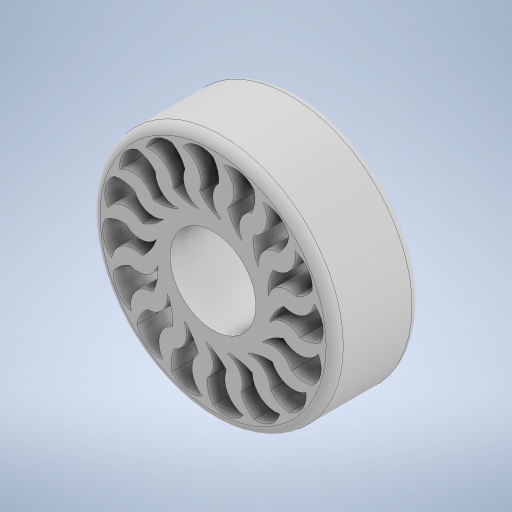
# Autodesk Inventor part: Idea1
Saved by Autodesk Inventor 2024.2 (Build 282272000, 272)
## iProperties
Created: 2025-06-20
Part Number: Idea1
Material: Generic
Document SubType Name: Modeling
Designer: Admin
Density: 1 g/cm^3
Appearance: Default
Author: Admin
Autodesk Inventor part; units mm, degrees
ref_plane "YZ Plane" through (0, 0, 0) normal (1, 0, 0) x (0, 1, 0)
ref_plane "XZ Plane" through (0, 0, 0) normal (0, 1, 0) x (-1, 0, 0)
ref_plane "XY Plane" through (0, 0, 0) normal (0, 0, 1) x (1, 0, 0)
sketch "Sketch1" plane through (0, 0, 0) normal (0, 0, 1) x (1, 0, 0)
  circle A0 centre (0, 0) radius 15
  circle A1 centre (0, 0) radius 42.5
  line L0 (2.6765, 14.7593) -> (2.6765, 19.7593) construction
  line L1 (0, 42.5) -> (0, 37.5) construction
  arc A2 (-4.6542, 24.6527) -> (2.6765, 19.7593) centre (7.5549, 35.0052) ccw
  arc A3 (-4.6542, 24.6527) -> (-10.5902, 35.3985) centre (-12.0817, 27.5622) ccw
  arc A4 (0, 37.5) -> (-10.5902, 35.3985) centre (-4.0532, 30.1908) ccw
  arc A5 (1.9949, 30.4737) -> (0, 37.5) centre (-8.5267, 31.2827) ccw
  arc A6 (1.9949, 30.4737) -> (2.6765, 19.7593) centre (7.0242, 25.4148) ccw
  arc A7 (-14.3506, 34.6455) -> (-23.3305, 28.6513) centre (-15.2982, 26.3416) ccw
  arc A8 (-13.7341, 20.995) -> (-23.3305, 28.6513) centre (-21.7096, 20.8406) ccw
  arc A9 (-9.8187, 28.9175) -> (-14.3506, 34.6455) centre (-19.849, 25.6385) ccw
  arc A10 (-9.8187, 28.9175) -> (-5.0888, 19.2795) centre (-3.2363, 26.1682) ccw
  arc A11 (-13.7341, 20.995) -> (-5.0888, 19.2795) centre (-6.4161, 35.2317) ccw
  arc A12 (-26.5165, 26.5165) -> (-32.5189, 17.5421) centre (-24.2141, 18.4821) ccw
  arc A13 (-20.7231, 14.141) -> (-32.5189, 17.5421) centre (-28.0324, 10.9463) ccw
  arc A14 (-20.1376, 22.9588) -> (-26.5165, 26.5165) centre (-28.1495, 16.091) ccw
  arc A15 (-20.1376, 22.9588) -> (-12.0793, 15.8645) centre (-13.0041, 22.9378) ccw
  arc A16 (-20.7231, 14.141) -> (-12.0793, 15.8645) centre (-19.4103, 30.0946) ccw
  arc A17 (-34.6455, 14.3506) -> (-36.7567, 3.7623) centre (-29.4437, 7.8089) ccw
  arc A18 (-24.5572, 5.1342) -> (-36.7567, 3.7623) centre (-30.0876, -0.6144) ccw
  arc A19 (-27.3906, 13.5049) -> (-34.6455, 14.3506) centre (-32.1645, 4.0938) ccw
  arc A20 (-27.3906, 13.5049) -> (-17.2309, 10.0343) centre (-20.7921, 16.2153) ccw
  arc A21 (-24.5572, 5.1342) -> (-17.2309, 10.0343) centre (-29.4495, 20.3757) ccw
  arc A22 (-37.5, 0) -> (-35.3985, -10.5902) centre (-30.1908, -4.0532) ccw
  arc A23 (-24.6527, -4.6542) -> (-35.3985, -10.5902) centre (-27.5622, -12.0817) ccw
  arc A24 (-30.4737, 1.9949) -> (-37.5, 0) centre (-31.2827, -8.5267) ccw
  arc A25 (-30.4737, 1.9949) -> (-19.7593, 2.6765) centre (-25.4148, 7.0242) ccw
  arc A26 (-24.6527, -4.6542) -> (-19.7593, 2.6765) centre (-35.0052, 7.5549) ccw
  arc A27 (-34.6455, -14.3506) -> (-28.6513, -23.3305) centre (-26.3416, -15.2982) ccw
  arc A28 (-20.995, -13.7341) -> (-28.6513, -23.3305) centre (-20.8406, -21.7096) ccw
  arc A29 (-28.9175, -9.8187) -> (-34.6455, -14.3506) centre (-25.6385, -19.849) ccw
  arc A30 (-28.9175, -9.8187) -> (-19.2795, -5.0888) centre (-26.1682, -3.2363) ccw
  arc A31 (-20.995, -13.7341) -> (-19.2795, -5.0888) centre (-35.2317, -6.4161) ccw
  arc A32 (-26.5165, -26.5165) -> (-17.5421, -32.5189) centre (-18.4821, -24.2141) ccw
  arc A33 (-14.141, -20.7231) -> (-17.5421, -32.5189) centre (-10.9463, -28.0324) ccw
  arc A34 (-22.9588, -20.1376) -> (-26.5165, -26.5165) centre (-16.091, -28.1495) ccw
  arc A35 (-22.9588, -20.1376) -> (-15.8645, -12.0793) centre (-22.9378, -13.0041) ccw
  arc A36 (-14.141, -20.7231) -> (-15.8645, -12.0793) centre (-30.0946, -19.4103) ccw
  arc A37 (-14.3506, -34.6455) -> (-3.7623, -36.7567) centre (-7.8089, -29.4437) ccw
  arc A38 (-5.1342, -24.5572) -> (-3.7623, -36.7567) centre (0.6144, -30.0876) ccw
  arc A39 (-13.5049, -27.3906) -> (-14.3506, -34.6455) centre (-4.0938, -32.1645) ccw
  arc A40 (-13.5049, -27.3906) -> (-10.0343, -17.2309) centre (-16.2153, -20.7921) ccw
  arc A41 (-5.1342, -24.5572) -> (-10.0343, -17.2309) centre (-20.3757, -29.4495) ccw
  arc A42 (0, -37.5) -> (10.5902, -35.3985) centre (4.0532, -30.1908) ccw
  arc A43 (4.6542, -24.6527) -> (10.5902, -35.3985) centre (12.0817, -27.5622) ccw
  arc A44 (-1.9949, -30.4737) -> (0, -37.5) centre (8.5267, -31.2827) ccw
  arc A45 (-1.9949, -30.4737) -> (-2.6765, -19.7593) centre (-7.0242, -25.4148) ccw
  arc A46 (4.6542, -24.6527) -> (-2.6765, -19.7593) centre (-7.5549, -35.0052) ccw
  arc A47 (14.3506, -34.6455) -> (23.3305, -28.6513) centre (15.2982, -26.3416) ccw
  arc A48 (13.7341, -20.995) -> (23.3305, -28.6513) centre (21.7096, -20.8406) ccw
  arc A49 (9.8187, -28.9175) -> (14.3506, -34.6455) centre (19.849, -25.6385) ccw
  arc A50 (9.8187, -28.9175) -> (5.0888, -19.2795) centre (3.2363, -26.1682) ccw
  arc A51 (13.7341, -20.995) -> (5.0888, -19.2795) centre (6.4161, -35.2317) ccw
  arc A52 (26.5165, -26.5165) -> (32.5189, -17.5421) centre (24.2141, -18.4821) ccw
  arc A53 (20.7231, -14.141) -> (32.5189, -17.5421) centre (28.0324, -10.9463) ccw
  arc A54 (20.1376, -22.9588) -> (26.5165, -26.5165) centre (28.1495, -16.091) ccw
  arc A55 (20.1376, -22.9588) -> (12.0793, -15.8645) centre (13.0041, -22.9378) ccw
  arc A56 (20.7231, -14.141) -> (12.0793, -15.8645) centre (19.4103, -30.0946) ccw
  arc A57 (34.6455, -14.3506) -> (36.7567, -3.7623) centre (29.4437, -7.8089) ccw
  arc A58 (24.5572, -5.1342) -> (36.7567, -3.7623) centre (30.0876, 0.6144) ccw
  arc A59 (27.3906, -13.5049) -> (34.6455, -14.3506) centre (32.1645, -4.0938) ccw
  arc A60 (27.3906, -13.5049) -> (17.2309, -10.0343) centre (20.7921, -16.2153) ccw
  arc A61 (24.5572, -5.1342) -> (17.2309, -10.0343) centre (29.4495, -20.3757) ccw
  arc A62 (37.5, 0) -> (35.3985, 10.5902) centre (30.1908, 4.0532) ccw
  arc A63 (24.6527, 4.6542) -> (35.3985, 10.5902) centre (27.5622, 12.0817) ccw
  arc A64 (30.4737, -1.9949) -> (37.5, 0) centre (31.2827, 8.5267) ccw
  arc A65 (30.4737, -1.9949) -> (19.7593, -2.6765) centre (25.4148, -7.0242) ccw
  arc A66 (24.6527, 4.6542) -> (19.7593, -2.6765) centre (35.0052, -7.5549) ccw
  arc A67 (34.6455, 14.3506) -> (28.6513, 23.3305) centre (26.3416, 15.2982) ccw
  arc A68 (20.995, 13.7341) -> (28.6513, 23.3305) centre (20.8406, 21.7096) ccw
  arc A69 (28.9175, 9.8187) -> (34.6455, 14.3506) centre (25.6385, 19.849) ccw
  arc A70 (28.9175, 9.8187) -> (19.2795, 5.0888) centre (26.1682, 3.2363) ccw
  arc A71 (20.995, 13.7341) -> (19.2795, 5.0888) centre (35.2317, 6.4161) ccw
  arc A72 (26.5165, 26.5165) -> (17.5421, 32.5189) centre (18.4821, 24.2141) ccw
  arc A73 (14.141, 20.7231) -> (17.5421, 32.5189) centre (10.9463, 28.0324) ccw
  arc A74 (22.9588, 20.1376) -> (26.5165, 26.5165) centre (16.091, 28.1495) ccw
  arc A75 (22.9588, 20.1376) -> (15.8645, 12.0793) centre (22.9378, 13.0041) ccw
  arc A76 (14.141, 20.7231) -> (15.8645, 12.0793) centre (30.0946, 19.4103) ccw
  arc A77 (14.3506, 34.6455) -> (3.7623, 36.7567) centre (7.8089, 29.4437) ccw
  arc A78 (5.1342, 24.5572) -> (3.7623, 36.7567) centre (-0.6144, 30.0876) ccw
  arc A79 (13.5049, 27.3906) -> (14.3506, 34.6455) centre (4.0938, 32.1645) ccw
  arc A80 (13.5049, 27.3906) -> (10.0343, 17.2309) centre (16.2153, 20.7921) ccw
  arc A81 (5.1342, 24.5572) -> (10.0343, 17.2309) centre (20.3757, 29.4495) ccw
  dimension "d0" = 30
  dimension "d1" = 85
  dimension "d2" = 5
  dimension "d3" = 5
  dimension "d6" = 360
  constraints: 160 point on circle, 80 centre point, 4 end point, 2 coincident, 2 vertical, 1 vertical alignment, 246 other
  measures "d2" distance of L0.start L0.end
  measures "d3" distance of L1.start L1.end
extrude "Extrusion1" add sketch "Sketch1" along normal blind 30
fillet "Fillet1" radius 3 2 edges at (-42.5, 0, 0) (-42.5, 0, 30)
body "Solid1"
